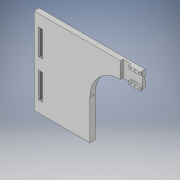
# Autodesk Inventor part: shoulder
Saved by Autodesk Inventor 2019 (Build 230136000, 136)
## iProperties
Created: 2018-10-19
Part Number: shoulder
Material: 일반
Document SubType Name: Modeling
Designer: otm09
Density: 1 g/cm^3
Appearance: 기본값
Author: otm09
Autodesk Inventor part; units mm, degrees
ref_plane "YZ Plane" through (0, 0, 0) normal (1, 0, 0) x (0, 1, 0)
ref_plane "XZ Plane" through (0, 0, 0) normal (0, 1, 0) x (-1, 0, 0)
ref_plane "XY Plane" through (0, 0, 0) normal (0, 0, 1) x (1, 0, 0)
sketch "스케치1" plane through (0, 0, 0) normal (0, 0, 1) x (1, 0, 0)
  line L0 (0, 0) -> (-110, 0)
  line L1 (-110, 0) -> (-110, -170)
  line L2 (-110, -170) -> (0, -170)
  line L3 (0, -170) -> (0, 0)
  line L4 (0, -40) -> (0, 0)
  line L5 (0, 0) -> (100, 0)
  line L6 (100, 0) -> (100, -32)
  line L7 (100, -32) -> (0, -32)
  line L8 (0, -32) -> (0, 0)
  line L9 (100, -5.5) -> (76, -5.5)
  line L10 (76, -5.5) -> (76, -26.5)
  line L11 (76, -26.5) -> (100, -26.5)
  line L12 (100, -26.5) -> (100, -5.5)
  circle A0 centre (96, -2.5) radius 1.1
  circle A1 centre (88, -2.5) radius 1.1
  circle A2 centre (80, -2.5) radius 1.1
  circle A3 centre (96, -29.5) radius 1.1
  circle A4 centre (88, -29.5) radius 1.1
  circle A5 centre (80, -29.5) radius 1.1
  line L13 (76, 0) -> (76, -5.5)
  line L14 (76, -26.5) -> (76, -32)
  line L15 (0, 0) -> (60, 0)
  line L16 (60, 0) -> (60, -32)
  line L17 (60, -32) -> (0, -32)
  line L18 (0, -32) -> (0, 0)
  line L19 (0, 0) -> (60, 0)
  line L20 (60, 0) -> (60, -32)
  line L21 (60, -32) -> (0, -32)
  line L22 (0, -32) -> (0, 0)
  dimension "d0" = 110
  dimension "d1" = 170
  dimension "d15" = 100
  dimension "d16" = 32
  dimension "d17" = 24
  dimension "d18" = 21
  dimension "d19" = 5.5
  dimension "d20" = 2.2
  dimension "d23" = 8
  dimension "d29" = 2.5
  dimension "d30" = 4
  dimension "d31" = 2.2
  dimension "d34" = 8
  dimension "d39" = 4
  dimension "d40" = 2.5
  dimension "d48" = 60
  constraints: 46 end point, 10 parallel, 7 horizontal, 6 centre point, 5 perpendicular, 5 point on line, 1 vertical, 8 other
  measures "d0" distance of L2.end L1.end
  measures "d1" distance of L1.end L0.end
  measures "d15" distance of L6.end L7.end
  measures "d16" distance of L5.end L6.end
  measures "d17" distance of L11.end L10.end
  measures "d18" distance of L10.end L9.end
  measures "d19" distance between parallel lines of L7 L11
  measures "d20" diameter of A0
  measures "d23" distance of A0.centre A1.centre
  measures "d29" distance from line of A0.centre L5
  measures "d30" distance from line of A0.centre L6
  measures "d31" diameter of A3
  measures "d34" distance of A3.centre A4.centre
  measures "d39" distance from line of A3.centre L6
  measures "d40" distance from line of L7 A3.centre
  measures "d48" distance of L16.end L17.end
extrude "돌출1" add sketch "스케치1" along normal blind 5.2 contours L3 L2 L1 L0 | L5 L16 L7 L3 | L5 L6 L9 L13 | L14 L11 L6 L7
extrude "돌출2" add sketch "스케치1" against normal blind 5
sketch "스케치2" plane through (0, 0, -5) normal (0, 0, -1) x (-1, 0, 0)
  circle A0 centre (-110.5, -16) radius 13
  circle A1 centre (-96, -2.5) radius 1.1 projected
  line L0 (-100, -32) -> (0, -32) projected
  line L1 (-100, 0) -> (-76, 0) projected
  line L2 (-76, -32) -> (-100, -32) projected
  line L3 (-100, 0) -> (-98.5, 0)
  line L4 (-98.5, 0) -> (-98.5, -32)
  line L5 (-98.5, -32) -> (-100, -32)
  line L6 (-100, -32) -> (-100, 0)
  point P0 (0, 0)
  dimension "d43" = 26
  dimension "d44" = 14.5
  dimension "d45" = 16
  dimension "d67" = 1.5
  constraints: 8 end point, 2 parallel, 1 centre point, 1 horizontal, 1 perpendicular, 1 point on line
  measures "d43" diameter of A0
  measures "d44" horizontal distance of A1.centre A0.centre
  measures "d45" distance from line of A0.centre L0
  measures "d67" distance of L4.end L5.end
extrude "돌출3" cut sketch "스케치2" against normal blind 5 contours A0 L4 | L4 A0 L6 | A0 L6 L1 L4 | L4 L0 L6 A0 | L6 A0
sketch "스케치3" plane through (0, 0, -5) normal (0, 0, -1) x (-1, 0, 0)
  circle A0 centre (-80, -29.5) radius 1.1 projected
  circle A1 centre (-80, -29.5) radius 2.1
  circle A2 centre (-88, -29.5) radius 1.1 projected
  circle A3 centre (-88, -29.5) radius 2.1
  circle A4 centre (-96, -29.5) radius 1.1 projected
  circle A5 centre (-96, -29.5) radius 2.1
  circle A6 centre (-80, -2.5) radius 1.1 projected
  circle A7 centre (-80, -2.5) radius 2.1
  circle A8 centre (-88, -2.5) radius 1.1 projected
  circle A9 centre (-88, -2.5) radius 2.1
  circle A10 centre (-96, -2.5) radius 1.1 projected
  circle A11 centre (-96, -2.5) radius 2.1
  point P0 (0, 0)
  dimension "d49" = 4.2
  dimension "d50" = 4.2
  dimension "d51" = 4.2
  dimension "d52" = 4.2
  dimension "d53" = 4.2
  dimension "d54" = 4.2
  constraints: 6 centre point, 6 coincident
  measures "d49" diameter of A1
  measures "d50" diameter of A3
  measures "d51" diameter of A5
  measures "d52" diameter of A7
  measures "d53" diameter of A9
  measures "d54" diameter of A11
extrude "돌출4" cut sketch "스케치3" against normal blind 8.2
fillet "모깎기2" radius 60 1 edges at (0, -32, 0.1)
sketch "스케치4" plane through (0, 0, 5.2) normal (0, 0, 1) x (1, 0, 0)
  line L0 (-100, -23.3333) -> (-95, -23.3333)
  line L1 (-95, -23.3333) -> (-95, -73.3333)
  line L2 (-95, -73.3333) -> (-100, -73.3333)
  line L3 (-100, -73.3333) -> (-100, -23.3333)
  line L4 (-100, -96.6667) -> (-95, -96.6667)
  line L5 (-95, -96.6667) -> (-95, -146.6667)
  line L6 (-95, -146.6667) -> (-100, -146.6667)
  line L7 (-100, -146.6667) -> (-100, -96.6667)
  line L8 (60, 0) -> (-110, 0) projected
  line L9 (-110, 0) -> (-110, -170) projected
  point P0 (0, 0)
  dimension "d58" = 5
  dimension "d59" = 50
  dimension "d60" = 5
  dimension "d61" = 50
  dimension "d62" = 23.3333
  dimension "d63" = 23.3333
  dimension "d64" = 10
  constraints: 16 end point, 4 parallel, 2 horizontal, 2 perpendicular, 1 point on line
  measures "d58" distance of L1.end L2.end
  measures "d59" distance of L0.end L1.end
  measures "d60" distance of L5.end L6.end
  measures "d61" distance of L4.end L5.end
  measures "d62" distance between parallel lines of L0 L8
  measures "d63" distance from line of L4.end L2
  measures "d64" distance between parallel lines of L3 L9
extrude "돌출5" cut sketch "스케치4" against normal blind 10.2
chamfer "모따기1" distance 3 distance2 1.5 1 edges at (100, -29.25, 0) measured on face at (100, -28.3333, 1.7333)
chamfer "모따기2" distance 3 distance2 1.5 1 edges at (100, -2.75, 0) measured on face at (100, -3.6667, 3.4667)
fillet "모깎기3" radius 2 8 edges at (-95, -48.3333, 5.2) (-100, -48.3333, 5.2) (-95, -121.6667, 5.2) (-100, -121.6667, 5.2) (-100, -121.6667, -5) (-95, -121.6667, -5) (-95, -48.3333, -5) (-100, -48.3333, -5)
equation "\"d19\" = -0.5 * d18 + 0.5 * d16"
